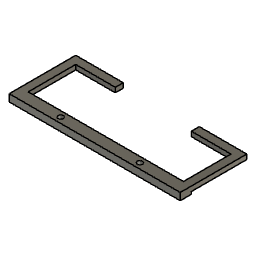
t265mount (Autodesk Fusion 360 design; units mm, degrees)
Autodesk Fusion 360 part; units mm, degrees
note: some values were not read from the file. Set by a fixed rule: which sketch regions a step uses.
sketch "Sketch1" plane through (0, 0, 0) normal (0, 0, 1) x (1, 0, 0)
  line L0 (54, 3.5) -> (-54, 3.5)
  line L1 (-54, 3.5) -> (-54, -3.5)
  line L2 (-54, -3.5) -> (54, -3.5)
  line L3 (54, -3.5) -> (54, 3.5)
  line L4 (54, 3.5) -> (-54, -3.5) construction
  line L5 (-54, 3.5) -> (54, -3.5) construction
  circle A0 centre (-25, 0) radius 1.675
  line L6 (0, 3.5) -> (0, -3.5) construction
  circle A1 centre (25, 0) radius 1.675
  dimension "d1" = 108
  dimension "width" = 7
  dimension "d3" = 3.35
  dimension "d21" = 25
  constraint horizontal L0
  constraint perpendicular L0 L1
  constraint parallel L0 L2
  constraint parallel L1 L3
  constraint coincident L4 origin
  constraint coincident L5 origin
  constraint midpoint L0 L6.start
  constraint midpoint L2 L6.end
  constraint symmetric A0 L6 A1
  measures "d1" distance of L1.end L2.end
  measures "width" distance of L0.end L1.end
  measures "d3" diameter of A0
  measures "d21" distance of A0.centre L6
extrude "Extrude1" add sketch "Sketch1" along normal blind 4.5
sketch "Sketch2" plane through (0, 3.5, 0) normal (0, 1, 0) x (-1, 0, 0)
  line L0 (-54, 0) -> (54, 0)
  line L1 (54, 0) -> (54, 4.5)
  line L2 (54, 4.5) -> (-54, 4.5)
  line L3 (-54, 4.5) -> (-54, 0)
  line L4 (-54, 4.5) -> (-49, 4.5)
  line L5 (-49, 4.5) -> (-49, 1.5)
  line L6 (-49, 1.5) -> (-54, 1.5)
  line L7 (-54, 1.5) -> (-54, 4.5)
  line L8 (0, 4.5) -> (0, 0) construction
  line L9 (49, 4.5) -> (49, 1.5)
  line L10 (49, 1.5) -> (54, 1.5)
  line L11 (54, 1.5) -> (54, 4.5)
  line L12 (54, 4.5) -> (49, 4.5)
  dimension "d6" = 5
  constraint horizontal L4
  constraint vertical L5
  constraint horizontal L6
  constraint vertical L7
  constraint coincident L2.end L3.start
  constraint midpoint L2 L8.start
  constraint coincident L8.end origin
  constraint symmetric L2.end L8 L1.end
  constraint symmetric L4.end L8 L9.start
  constraint symmetric L5.end L8 L9.end
  constraint symmetric L6.end L8 L10.end
  measures "d6" distance of L2.end L4.end
extrude "Extrude2" add sketch "Sketch2" along normal blind 35 contours L2 L3 L4 L5 L6 L7 | L1 L2 L9 L10 L11 L12
sketch "Sketch3" plane through (-49, 0, 0) normal (1, 0, 0) x (0, 1, 0)
  line L0 (3.5, 4.5) -> (3.5, 1.5)
  line L1 (3.5, 1.5) -> (38.5, 1.5)
  line L2 (38.5, 1.5) -> (38.5, 4.5)
  line L3 (38.5, 4.5) -> (3.5, 4.5)
  line L4 (38.5, 4.5) -> (33.5, 4.5)
  line L5 (33.5, 4.5) -> (33.5, 1.5)
  line L6 (33.5, 1.5) -> (38.5, 1.5)
  line L7 (38.5, 1.5) -> (38.5, 4.5)
  dimension "d9" = 5
  constraint horizontal L4
  constraint vertical L5
  constraint horizontal L6
  constraint vertical L7
  constraint coincident L2.end L3.start
  measures "d9" distance of L2.end L4.end
sketch "Sketch4" plane through (49, 0, 0) normal (-1, 0, 0) x (0, -1, 0)
  line L0 (-3.5, 1.5) -> (-3.5, 4.5)
  line L1 (-3.5, 4.5) -> (-38.5, 4.5)
  line L2 (-38.5, 4.5) -> (-38.5, 1.5)
  line L3 (-38.5, 1.5) -> (-3.5, 1.5)
  line L4 (-38.5, 4.5) -> (-33.5, 4.5)
  line L5 (-33.5, 4.5) -> (-33.5, 1.5)
  line L6 (-33.5, 1.5) -> (-38.5, 1.5)
  line L7 (-38.5, 1.5) -> (-38.5, 4.5)
  dimension "d10" = 5
  constraint horizontal L4
  constraint vertical L5
  constraint horizontal L6
  constraint vertical L7
  constraint coincident L1.end L2.start
  measures "d10" distance of L1.end L4.end
extrude "Extrude3" add sketch "Sketch4" along normal blind 25 contours L1 L2 L3 L4 L5 L6 L7
extrude "Extrude4" add sketch "Sketch3" along normal blind 25 contours L1 L2 L3 L4 L5 L6 L7
sketch "Sketch5" plane through (0, 0, 4.5) normal (0, 0, 1) x (-1, 0, 0)
  circle A0 centre (25, 0) radius 1.675
  circle A1 centre (-25, 0) radius 1.675
  line L0 (-54, 3.5) -> (-54, -38.5)
  line L1 (-54, -38.5) -> (-24, -38.5)
  line L2 (-24, -38.5) -> (-24, -33.5)
  line L3 (-24, -33.5) -> (-49, -33.5)
  line L4 (-49, -33.5) -> (-49, -3.5)
  line L5 (-49, -3.5) -> (49, -3.5)
  line L6 (49, -3.5) -> (49, -33.5)
  line L7 (49, -33.5) -> (24, -33.5)
  line L8 (24, -33.5) -> (24, -38.5)
  line L9 (24, -38.5) -> (54, -38.5)
  line L10 (54, -38.5) -> (54, 3.5)
  line L11 (54, 3.5) -> (-54, 3.5)
  line L12 (-24, -36) -> (-54, -36) construction
  constraint midpoint L2 L12.start
  constraint coincident L0 L12.end
  constraint perpendicular L0 L12
extrude "Extrude5" [suppressed]
